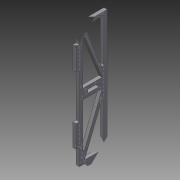
# Autodesk Inventor part: Battery holder
Saved by Autodesk Inventor 2015 (Build 190159000, 159)
## iProperties
Created: 2014-08-15
Part Number: Battery holder
Material: Generic
Document SubType Name: Modeling
Designer: karl
Density: 1 g/cm^3
Appearance: Default
Author: karl
Autodesk Inventor part; units mm, degrees
ref_plane "YZ Plane" through (0, 0, 0) normal (1, 0, 0) x (0, 1, 0)
ref_plane "XZ Plane" through (0, 0, 0) normal (0, 1, 0) x (-1, 0, 0)
ref_plane "XY Plane" through (0, 0, 0) normal (0, 0, 1) x (1, 0, 0)
sketch "Sketch1" plane through (0, 0, 0) normal (1, 0, 0) x (0, 1, 0)
  line L0 (-12.5, -55) -> (12.5, -55)
  line L1 (12.5, -55) -> (12.5, 55)
  line L2 (12.5, 55) -> (-12.5, 55)
  line L3 (-12.5, 55) -> (-12.5, -55)
  line L4 (-12.5, -55) -> (12.5, 55) construction
  line L5 (12.5, -55) -> (-12.5, 55) construction
  point P0 (0, 0)
  dimension "d0" = 25
  dimension "d1" = 110
  constraints: 12 end point, 2 midpoint, 2 parallel, 1 horizontal, 1 perpendicular
  measures "d0" distance of L2.end L1.end
  measures "d1" distance of L1.end L0.end
extrude "Extrusion1" add sketch "Sketch1" along normal blind 3
sketch "Sketch2" plane through (3, 0, 0) normal (1, 0, 0) x (0, 0, -1)
  line L0 (20, -12.5) -> (40, -12.5)
  line L1 (40, -12.5) -> (40, -15.5)
  line L2 (40, -15.5) -> (20, -15.5)
  line L3 (20, -15.5) -> (20, -12.5)
  line L4 (-55, -12.5) -> (55, -12.5) projected
  line L5 (-20, -12.5) -> (-40, -12.5)
  line L6 (-40, -12.5) -> (-40, -15.5)
  line L7 (-40, -15.5) -> (-20, -15.5)
  line L8 (-20, -15.5) -> (-20, -12.5)
  point P0 (0, 0)
  dimension "d4" = 20
  dimension "d5" = 3
  dimension "d6" = 20
  dimension "d7" = 20
  dimension "d8" = 3
  dimension "d9" = 20
  constraints: 16 end point, 4 parallel, 2 horizontal, 2 perpendicular, 1 collinear, 1 point on line
  measures "d4" distance of L1.end L2.end
  measures "d5" distance of L0.end L1.end
  measures "d6" distance from line of L3 point (0, 0)
  measures "d7" distance of L7.end L6.end
  measures "d8" distance of L6.end L5.end
  measures "d9" distance from line of point (0, 0) L8
extrude "Extrusion2" add sketch "Sketch2" against normal blind 3
sketch "Sketch3" plane through (3, 0, 0) normal (1, 0, 0) x (0, 0, -1)
  line L0 (-1.5, 5) -> (1.5, 5)
  line L1 (1.5, 5) -> (1.5, -5)
  line L2 (1.5, -5) -> (-1.5, -5)
  line L3 (-1.5, -5) -> (-1.5, 5)
  point P0 (0, 0)
  point P1 (-1.5, 0)
  point P2 (0, 5)
  dimension "d12" = 3
  dimension "d13" = 10
  constraints: 8 end point, 2 midpoint, 2 parallel, 1 horizontal, 1 horizontal alignment, 1 perpendicular, 1 vertical alignment
  measures "d12" distance of L1.end L2.end
  measures "d13" distance of L0.end L1.end
extrude "Extrusion3" cut sketch "Sketch3" against normal blind 3
sketch "Sketch4" plane through (3, 0, 0) normal (1, 0, 0) x (0, 0, -1)
  line L0 (55, -12.5) -> (55, 12.5) projected
  line L1 (55, 5) -> (58, 5)
  line L2 (58, 5) -> (58, -5)
  line L3 (58, -5) -> (55, -5)
  line L4 (55, -5) -> (55, 5)
  point P0 (0, 0)
  point P1 (58, 0)
  point P2 (55, 0)
  dimension "d16" = 3
  dimension "d17" = 10
  constraints: 8 end point, 2 midpoint, 2 parallel, 1 horizontal, 1 horizontal alignment, 1 perpendicular, 1 point on line
  measures "d16" distance of L2.end L3.end
  measures "d17" distance of L1.end L2.end
extrude "Extrusion4" add sketch "Sketch4" against normal blind 3
sketch "Sketch5" plane through (3, 0, 0) normal (1, 0, 0) x (0, 0, -1)
  line L0 (4.5, 9.5) -> (52, 9.5)
  line L1 (52, 9.5) -> (52, -9.5)
  line L2 (52, -9.5) -> (4.5, -9.5)
  line L3 (4.5, -9.5) -> (4.5, 9.5)
  line L4 (55, 12.5) -> (-55, 12.5) projected
  line L5 (1.5, -5) -> (1.5, 5) projected
  line L6 (55, 5) -> (55, 12.5) projected
  line L7 (40, -12.5) -> (55, -12.5) projected
  point P0 (0, 0)
  dimension "d20" = 3
  dimension "d21" = 3
  dimension "d22" = 3
  dimension "d23" = 3
  constraints: 8 end point, 2 parallel, 1 horizontal, 1 perpendicular
  measures "d20" distance between parallel lines of L4 L0
  measures "d21" distance between parallel lines of L5 L3
  measures "d22" distance between parallel lines of L6 L1
  measures "d23" distance between parallel lines of L7 L2
extrude "Extrusion5" cut sketch "Sketch5" against normal blind 3
sketch "Sketch6" plane through (3, 0, 0) normal (1, 0, 0) x (0, 0, -1)
  line L0 (4.5, 9.5) -> (52, -9.5) construction
  line L1 (3.9429, 8.1073) -> (51.4429, -10.8927)
  line L2 (52.5571, -8.1073) -> (5.0571, 10.8927)
  arc A0 (5.0571, 10.8927) -> (3.9429, 8.1073) centre (4.5, 9.5) ccw
  arc A1 (51.4429, -10.8927) -> (52.5571, -8.1073) centre (52, -9.5) ccw
  point P0 (0, 0)
  point P1 (28.25, 0)
  dimension "d26" = 3
  constraints: 8 end point, 4 point on circle, 4 tangent, 2 centre point, 1 midpoint, 1 parallel
  measures "d26" diameter of A1
extrude "Extrusion6" add sketch "Sketch6" against normal blind 3
fillet "Fillet1" radius 1 2 edges at (1.5, -9.5, -47.9611) (1.5, 9.5, -8.5389)
mirror "Mirror1" about plane through (0, 0, 0) normal (0, 0, 1) of "Extrusion5", "Extrusion6", "Fillet1", "Extrusion4"
equation "\"d9\" = d6"
equation "\"d23\" = d20"
body "Solid1"
